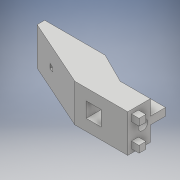
# Autodesk Inventor part: end
Saved by Autodesk Inventor 2017 (Build 210142000, 142)
## iProperties
Created: 2017-03-24
Part Number: end
Material: Generic
Document SubType Name: Modeling
Designer: PC
Density: 1 g/cm^3
Appearance: Default
Author: PC
Autodesk Inventor part; units mm, degrees
ref_plane "YZ Plane" through (0, 0, 0) normal (1, 0, 0) x (0, 1, 0)
ref_plane "XZ Plane" through (0, 0, 0) normal (0, 1, 0) x (-1, 0, 0)
ref_plane "XY Plane" through (0, 0, 0) normal (0, 0, 1) x (1, 0, 0)
sketch "Sketch1" plane through (0, 0, 0) normal (1, 0, 0) x (0, 1, 0)
  line L0 (-7.5, -12.5) -> (7.5, -12.5)
  line L1 (7.5, -12.5) -> (7.5, 12.5)
  line L2 (7.5, 12.5) -> (-7.5, 12.5)
  line L3 (-7.5, 12.5) -> (-7.5, -12.5)
  line L4 (-7.5, -12.5) -> (7.5, 12.5) construction
  line L5 (7.5, -12.5) -> (-7.5, 12.5) construction
  point P0 (0, 0)
  dimension "d0" = 15
  dimension "d1" = 25
  constraints: 12 end point, 2 midpoint, 2 parallel, 1 horizontal, 1 perpendicular
  measures "d0" distance of L2.end L1.end
  measures "d1" distance of L1.end L0.end
extrude "Extrusion1" add sketch "Sketch1" against normal blind 80
sketch "Sketch2" plane through (0, 0, 0) normal (1, 0, 0) x (0, 0, -1)
  line L0 (-12.5, 7.5) -> (12.5, 7.5) projected
  line L1 (0, 7.5) -> (2.5, 7.5)
  line L2 (2.5, 7.5) -> (2.5, 17.5)
  line L3 (2.5, 17.5) -> (0, 17.5)
  line L4 (0, 17.5) -> (0, 7.5)
  line L5 (0, 7.5) -> (-2.5, 7.5)
  line L6 (-2.5, 7.5) -> (-2.5, 17.5)
  line L7 (-2.5, 17.5) -> (0, 17.5)
  line L8 (0, 17.5) -> (0, 7.5)
  point P0 (0, 0)
  dimension "d4" = 2.5
  dimension "d5" = 10
  dimension "d6" = 2.5
  dimension "d7" = 10
  constraints: 16 end point, 4 parallel, 2 horizontal, 2 perpendicular, 1 midpoint
  measures "d4" distance of L3.end L2.end
  measures "d5" distance of L2.end L1.end
  measures "d6" distance of L6.end L7.end
  measures "d7" distance of L5.end L6.end
extrude "Extrusion2" add sketch "Sketch2" against normal blind 80
sketch "Sketch4" plane through (0, 7.5, -2.5) normal (0, 0, -1) x (-1, 0, 0)
  line L0 (80, -15) -> (80, 0) projected
  line L1 (80, 0) -> (40, 0)
  line L2 (40, 0) -> (40, 10)
  line L3 (40, 10) -> (80, 10)
  line L4 (80, 10) -> (80, 0)
  point P0 (0, -7.5)
  dimension "d12" = 40
  constraints: 8 end point, 2 parallel, 1 horizontal, 1 perpendicular
  measures "d12" distance of L2.end L3.end
extrude "Extrusion3" add sketch "Sketch4" along normal blind 10
sketch "Sketch5" plane through (0, 7.5, -2.5) normal (0, 0, -1) x (-1, 0, 0)
  line L0 (0, 0) -> (80, 0) projected
  line L1 (40, 0) -> (20, 0)
  line L2 (20, 0) -> (40, 10)
  line L3 (40, 10) -> (40, 0)
  point P0 (0, -7.5)
  dimension "d15" = 20
  constraints: 6 end point, 1 midpoint, 1 perpendicular, 1 point on line
  measures "d15" distance of L1.start L1.end
extrude "Extrusion4" add sketch "Sketch5" along normal blind 10
sketch "Sketch6" plane through (0, 7.5, 2.5) normal (0, 0, 1) x (1, 0, 0)
  line L0 (-80, 10) -> (-40, 10)
  line L1 (-40, 10) -> (-40, 0)
  line L2 (-40, 0) -> (-80, 0)
  line L3 (-80, 0) -> (-80, 10)
  point P0 (0, -7.5)
  constraints: 8 end point, 2 parallel, 1 horizontal, 1 perpendicular
extrude "Extrusion5" add sketch "Sketch6" along normal blind 10
sketch "Sketch7" plane through (0, 7.5, 2.5) normal (0, 0, 1) x (1, 0, 0)
  line L0 (-40, 10) -> (-40, 0) projected
  line L1 (-40, 0) -> (-20, 0)
  line L2 (0, 0) -> (-40, 0) projected
  line L3 (0, 10) -> (-40, 10) projected
  line L4 (-20, 0) -> (-40, 10)
  line L5 (-40, 10) -> (-40, 0)
  point P0 (0, -7.5)
  dimension "d20" = 20
  constraints: 6 end point, 1 midpoint, 1 perpendicular
  measures "d20" distance of L0.end L1.end
extrude "Extrusion6" add sketch "Sketch7" along normal blind 10
sketch "Sketch8" plane through (0, -7.5, 12.5) normal (0, 0, 1) x (1, 0, 0)
  line L0 (0, 0) -> (-80, 0) projected
  line L1 (-80, 0) -> (-80, 20)
  line L2 (-80, 0) -> (-80, 25) projected
  line L3 (-80, 0) -> (-35, 0)
  line L4 (-35, 0) -> (-80, 20)
  point P0 (0, 7.5)
  dimension "d23" = 20
  dimension "d24" = 45
  constraints: 6 end point, 2 point on line
  measures "d23" distance of L0.end L1.end
  measures "d24" distance of L0.end L3.end
extrude "Extrusion7" cut sketch "Sketch8" against normal blind 25
sketch "Sketch21" plane through (0, 17.5, 2.5) normal (0, 1, 0) x (1, 0, 0)
  line L0 (-62.5195, 3.1) -> (-63.7195, 3.1)
  line L1 (-63.7195, 3.1) -> (-63.7195, 1.9)
  line L2 (-63.7195, 1.9) -> (-62.5195, 1.9)
  line L3 (-62.5195, 1.9) -> (-62.5195, 3.1)
  line L4 (-62.5195, 3.1) -> (-63.7195, 1.9) construction
  line L5 (-63.7195, 3.1) -> (-62.5195, 1.9) construction
  point P0 (0, 2.5)
  point P1 (-63.1195, 2.5)
  dimension "d63" = 1.2
  dimension "d64" = 1.2
  constraints: 12 end point, 2 midpoint, 2 parallel, 1 horizontal, 1 perpendicular
  measures "d63" distance of L2.end L1.end
  measures "d64" distance of L1.end L0.end
extrude "Extrusion15" cut sketch "Sketch21" against normal blind 8.2
sketch "Sketch28" plane through (0, -7.5, -12.5) normal (0, -1, 0) x (1, 0, 0)
  line L0 (-17.5, 7.5) -> (-27.5, 7.5)
  line L1 (-27.5, 7.5) -> (-27.5, 17.5)
  line L2 (-27.5, 17.5) -> (-17.5, 17.5)
  line L3 (-17.5, 17.5) -> (-17.5, 7.5)
  line L4 (-17.5, 7.5) -> (-27.5, 17.5) construction
  line L5 (-27.5, 7.5) -> (-17.5, 17.5) construction
  point P0 (0, 12.5)
  point P1 (-22.5, 12.5)
  dimension "d86" = 10
  dimension "d87" = 10
  constraints: 12 end point, 2 midpoint, 2 parallel, 1 horizontal, 1 perpendicular
  measures "d86" distance of L1.end L2.end
  measures "d87" distance of L0.end L1.end
extrude "Extrusion18" cut sketch "Sketch28" against normal blind 10
sketch "Sketch30" plane through (0, 0, 0) normal (1, 0, 0) x (0, 0, -1)
  line L0 (-12.5, -7.5) -> (12.5, -7.5) projected
  line L1 (0, -7.5) -> (0, 2.5)
  point P0 (0, 0)
  dimension "d90" = 10
  constraints: 2 end point, 1 midpoint, 1 vertical
  measures "d90" distance of L1.start L1.end
hole "Hole1" at (0, 2.5, 0) direction (-1, 0, 0) diameter 6.4 depth 10 tip angle 118
sketch "Sketch31" plane through (0, 9.3, 2.5) normal (0, 1, 0) x (1, 0, 0)
  line L0 (-64.5195, 1.1) -> (-61.7195, 1.1)
  line L1 (-61.7195, 1.1) -> (-61.7195, 3.9)
  line L2 (-61.7195, 3.9) -> (-64.5195, 3.9)
  line L3 (-64.5195, 3.9) -> (-64.5195, 1.1)
  line L4 (-64.5195, 1.1) -> (-61.7195, 3.9) construction
  line L5 (-61.7195, 1.1) -> (-64.5195, 3.9) construction
  point P0 (0, 2.5)
  point P1 (-63.1195, 2.5)
  dimension "d98" = 2.8
  dimension "d99" = 2.8
  constraints: 12 end point, 2 midpoint, 2 parallel, 1 horizontal, 1 perpendicular
  measures "d98" distance of L2.end L1.end
  measures "d99" distance of L1.end L0.end
extrude "Extrusion19" cut sketch "Sketch31" against normal through all
chamfer "Chamfer3" distance 0.8 angle 45 4 edges at (-62.5195, 9.3, 0) (-63.1195, 9.3, -0.6) (-63.1195, 9.3, 0.6) (-63.7195, 9.3, 0)
sketch "Sketch32" plane through (0, 0, 0) normal (1, 0, 0) x (0, 0, -1)
  line L0 (-12.5, -7.5) -> (12.5, -7.5) projected
  line L1 (-12.5, -7.5) -> (-10, -7.5)
  line L2 (-10, -7.5) -> (-10, -5)
  line L3 (-10, -5) -> (-12.5, -5)
  line L4 (-12.5, -5) -> (-12.5, -7.5)
  line L5 (-10, -5) -> (-5.5, -5)
  line L6 (-5.5, -5) -> (-5.5, -0.5)
  line L7 (-5.5, -0.5) -> (-10, -0.5)
  line L8 (-10, -0.5) -> (-10, -5)
  point P0 (0, 0)
  dimension "d105" = 2.5
  dimension "d106" = 2.5
  dimension "d107" = 4.5
  dimension "d108" = 4.5
  constraints: 16 end point, 4 parallel, 2 horizontal, 2 perpendicular
  measures "d105" distance of L3.end L2.end
  measures "d106" distance of L2.end L1.end
  measures "d107" distance of L7.end L6.end
  measures "d108" distance of L6.end L5.end
extrude "Extrusion20" add sketch "Sketch32" along normal blind 5 contours L8 L7 L6 L5
sketch "Sketch33" plane through (0, 0, 0) normal (1, 0, 0) x (0, 0, -1)
  line L0 (12.5, -7.5) -> (12.5, 12.5) projected
  line L1 (12.5, -7.5) -> (10, -7.5)
  line L2 (10, -7.5) -> (10, -5)
  line L3 (10, -5) -> (12.5, -5)
  line L4 (12.5, -5) -> (12.5, -7.5)
  line L5 (10, -5) -> (5.5, -5)
  line L6 (5.5, -5) -> (5.5, -0.5)
  line L7 (5.5, -0.5) -> (10, -0.5)
  line L8 (10, -0.5) -> (10, -5)
  point P0 (0, 0)
  dimension "d111" = 2.5
  dimension "d112" = 2.5
  dimension "d113" = 4.5
  dimension "d114" = 4.5
  constraints: 16 end point, 4 parallel, 2 horizontal, 2 perpendicular
  measures "d111" distance of L2.end L3.end
  measures "d112" distance of L1.end L2.end
  measures "d113" distance of L6.end L7.end
  measures "d114" distance of L5.end L6.end
extrude "Extrusion21" add sketch "Sketch33" along normal blind 5 contours L5 L6 L7 L8
body "Solid1"
